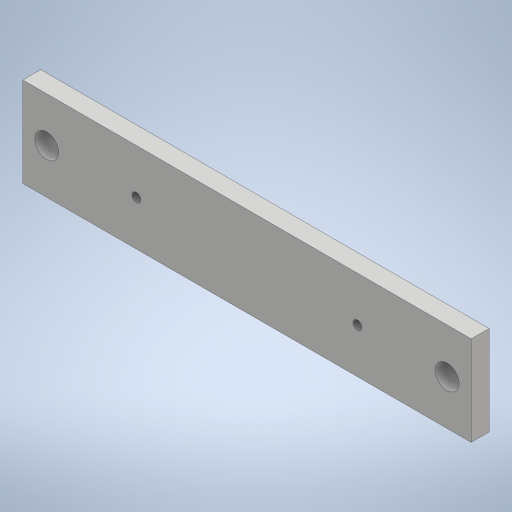
# Autodesk Inventor part: Soporte fuente
Saved by Autodesk Inventor 2024.2 (Build 282272000, 272)
## iProperties
Created: 2025-06-19
Part Number: Soporte fuente
Material: Genérico
Document SubType Name: Modeling
Designer: jd.castellanosq
Density: 1 g/cm^3
Appearance: Valor por defecto
Author: jd.castellanosq
Autodesk Inventor part; units mm, degrees
ref_plane "YZ Plane" through (0, 0, 0) normal (1, 0, 0) x (0, 1, 0)
ref_plane "XZ Plane" through (0, 0, 0) normal (0, 1, 0) x (-1, 0, 0)
ref_plane "XY Plane" through (0, 0, 0) normal (0, 0, 1) x (1, 0, 0)
sketch "Boceto1" plane through (0, 0, 0) normal (0, 1, 0) x (-1, 0, 0)
  line L0 (75, -15) -> (-75, -15)
  line L1 (-75, -15) -> (-75, 15)
  line L2 (-75, 15) -> (75, 15)
  line L3 (75, 15) -> (75, -15)
  circle A0 centre (-37, 0) radius 1.5
  circle A1 centre (37, 0) radius 1.5
  circle A2 centre (-67, 0) radius 4
  circle A3 centre (67, 0) radius 4
  point P0 (0, 0)
  point P1 (0, -15)
  point P2 (-75, 0)
  point P3 (75, 0)
  dimension "d0" = 30
  dimension "d1" = 150
  dimension "d6" = 3
  dimension "d7" = 8
  dimension "d8" = 8
  dimension "d9" = 8
  dimension "d16" = 74
  dimension "d17" = 37
  constraints: 8 end point, 5 horizontal alignment, 4 centre point, 3 midpoint, 2 equal radius, 2 parallel, 1 horizontal, 1 perpendicular, 1 vertical alignment
  measures "d0" distance of L0.end L1.end
  measures "d1" distance between parallel lines of L1 L3
  measures "d6" diameter of A0
  measures "d7" diameter of A3
  measures "d8" distance from line of A3.centre L3
  measures "d9" distance from line of L1 A2.centre
  measures "d16" distance of A0.centre A1.centre
  measures "d17" distance of A0.centre point (0, 0)
extrude "Extrusión1" add sketch "Boceto1" along normal blind 6
thread "Rosca1" size "M3x0.5" class "6H" standard "ANSI Metric M Profile" full length
thread "Rosca2" size "M3x0.5" class "6H" standard "ANSI Metric M Profile" full length
equation "\"d9\" = d8"
equation "\"d17\" = 0.5 * d16"
